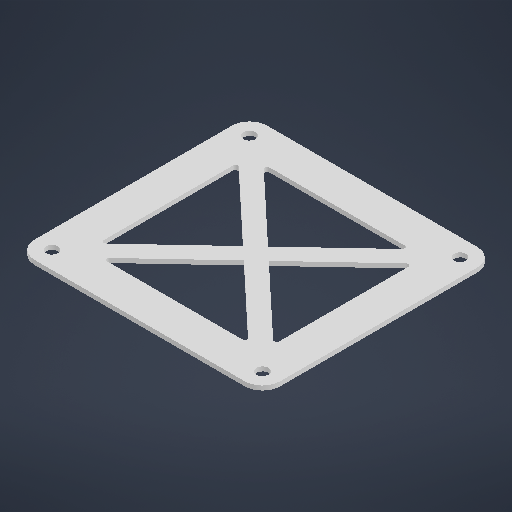
# Autodesk Inventor part: Hookcrossbrace
Saved by Autodesk Inventor 2025.2 (Build 292293000, 293)
## iProperties
Created: 2025-04-04
Part Number: Hookcrossbrace
Material: Generic
Document SubType Name: Modeling
Designer: Jahan
Density: 1 g/cm^3
Appearance: Default
Author: Jahan
Autodesk Inventor part; units mm, degrees
ref_plane "YZ Plane" through (0, 0, 0) normal (1, 0, 0) x (0, 1, 0)
ref_plane "XZ Plane" through (0, 0, 0) normal (0, 1, 0) x (-1, 0, 0)
ref_plane "XY Plane" through (0, 0, 0) normal (0, 0, 1) x (1, 0, 0)
sketch "Sketch1" plane through (0, 0, 0) normal (0, 1, 0) x (-1, 0, 0)
  circle A0 centre (-31.5089, -30.9076) radius 2.1844
  circle A1 centre (-31.5089, 40.6188) radius 2.1844
  circle A2 centre (44.6911, -30.9076) radius 2.1844
  circle A3 centre (44.6911, 40.6188) radius 2.1844
  circle A4 centre (44.6911, 40.6188) radius 6.35
  circle A5 centre (44.6911, -30.9076) radius 6.35
  circle A6 centre (-31.5089, -30.9076) radius 6.35
  circle A7 centre (-31.5089, 40.6188) radius 6.35
  line L0 (44.6911, 46.9688) -> (-31.5089, 46.9688)
  line L1 (-37.8589, 40.6188) -> (-37.8589, -30.9076)
  line L2 (-31.5089, -37.2576) -> (44.6911, -37.2576)
  line L3 (51.0411, -30.9076) -> (51.0411, 40.6188)
  line L4 (44.6911, 34.2688) -> (-31.5089, 34.2688)
  line L5 (-25.1589, 40.6188) -> (-25.1589, -30.9076)
  line L6 (-31.5089, -24.5576) -> (44.6911, -24.5576)
  line L7 (38.3411, 40.6188) -> (38.3411, -30.9076)
  line L8 (38.3411, 35.5878) -> (38.3411, 29.2378)
  line L9 (-25.1589, -24.5576) -> (-25.1589, -18.2076)
  line L10 (-25.1589, 34.2688) -> (-25.1589, 27.9188)
  line L11 (38.3411, -24.5576) -> (38.3411, -21.3826)
  line L12 (38.3411, -24.5576) -> (35.1661, -24.5576)
  line L13 (38.3411, 34.2688) -> (38.3411, 27.9188)
  line L14 (38.3411, -24.5576) -> (31.9911, -24.5576)
  circle A8 centre (-31.5089, 40.6188) radius 3.175
  circle A9 centre (44.6911, 40.6188) radius 3.175
  circle A10 centre (44.6911, -30.9076) radius 3.175
  circle A11 centre (-31.5089, -30.9076) radius 3.175
  line L15 (42.5182, 42.9337) -> (-33.6818, -28.5927)
  line L16 (46.8641, 38.3039) -> (-29.3359, -33.2225)
  line L17 (-29.3359, 42.9337) -> (46.8641, -28.5927)
  line L18 (-33.6818, 38.3039) -> (42.5182, -33.2225)
  arc A12 (31.6495, 32.7316) -> (31.041, 34.2688) centre (31.041, 33.3798) ccw
  arc A13 (38.3411, 28.2499) -> (36.8437, 28.8981) centre (37.4521, 28.2499) ccw
  arc A14 (36.8437, -19.1869) -> (38.3411, -18.5387) centre (37.4521, -18.5387) ccw
  arc A15 (31.041, -24.5576) -> (31.6495, -23.0204) centre (31.041, -23.6686) ccw
  arc A16 (-17.8588, 34.2688) -> (-18.4672, 32.7316) centre (-17.8588, 33.3798) ccw
  arc A17 (-23.6614, 28.8981) -> (-25.1589, 28.2499) centre (-24.2699, 28.2499) ccw
  arc A18 (-25.1589, -18.5387) -> (-23.6614, -19.1869) centre (-24.2699, -18.5387) ccw
  arc A19 (-18.4672, -23.0204) -> (-17.8588, -24.5576) centre (-17.8588, -23.6686) ccw
  point P0 (-25.1589, 30.3037)
  point P1 (1.952, 4.8556)
  point P2 (-25.1589, -20.5925)
  point P3 (-20.1048, 34.2688)
  point P4 (33.2871, 34.2688)
  point P5 (6.5911, 9.2102)
  point P6 (6.5911, 0.501)
  point P7 (-20.1048, -24.5576)
  point P8 (11.2303, 4.8556)
  point P9 (-25.1589, 28.2499)
  point P10 (-25.1589, -18.5387)
  dimension "d0" = 12.7
  dimension "d1" = 12.7
  dimension "d2" = 12.7
  dimension "d3" = 12.7
  dimension "d8" = 6.35
  dimension "d11" = 6.35
  dimension "d14" = 6.35
  dimension "d16" = 6.35
  dimension "d17" = 6.35
  dimension "d18" = 6.35
  dimension "d19" = 6.35
  dimension "d20" = 6.35
  dimension "d21" = 0.889
  dimension "d22" = 0.889
  dimension "d23" = 0.889
  dimension "d24" = 0.889
  dimension "d25" = 0.889
  dimension "d26" = 0.889
  dimension "d27" = 0.889
  dimension "d28" = 0.889
  constraints: 40 point on circle, 36 end point, 30 tangent, 24 point on line, 20 centre point, 8 coincident, 18 other
  measures "d0" diameter of A4
  measures "d1" diameter of A5
  measures "d2" diameter of A6
  measures "d3" diameter of A7
  measures "d8" distance of L9.start L9.end
  measures "d11" distance of L10.start L10.end
  measures "d14" distance of L13.start L13.end
  measures "d16" distance of L11.start L14.end
  measures "d17" diameter of A8
  measures "d18" diameter of A9
  measures "d19" diameter of A10
  measures "d20" diameter of A11
  measures "d21" radius of A12
  measures "d22" radius of A13
  measures "d23" radius of A14
  measures "d24" radius of A15
  measures "d25" radius of A16
  measures "d26" radius of A17
  measures "d27" radius of A18
  measures "d28" radius of A19
extrude "Extrusion1" add sketch "Sketch1" along normal blind 1.5875 contours A4 L16 A9 L15 | L3 A5 L6 L17 L7 L16 L4 A4 | A4 L7 L15 L4 L17 L5 A7 L0 | L4 L16 A4 | A5 L18 A10 L17 | A4 L15 L7 | A7 L17 A8 L18 | L16 L4 L7 L15 A4 | A4 L15 A9 L16 | L16 L7 L4 | A5 L17 L6 | L2 A6 L5 L16 L6 L18 L7 A5 | L7 L4 L15 | L5 L17 A7 | A7 L4 L18 L5 L15 L6 A6 L1 | A9 | L7 L16 L17 L15 L4 | L7 A13 L16 | L17 A10 L18 A5 | A5 L18 L7 L6 L17 | L6 L7 L17 | L7 L18 A5 | A6 L15 A11 L16 | L15 A12 L4 | L17 L5 L4 L18 A7 | A7 L18 A8 L17 | L17 L4 L5 | A7 L18 L4 | A10 | L7 L18 L6 | L6 L18 L16 L17 L7 | L17 A14 L7 | A6 L16 L5 | A8 | L5 L18 L4 | L4 L17 L15 L18 L5 | L4 A16 L17 | L6 L15 A6 | L16 L18 L15 L17 | L6 A15 L18 | L16 A11 L15 A6 | A6 L15 L6 L5 L16 | L5 L6 L16 | L18 A17 L5 | L15 L5 L6 | L16 L6 L5 L15 L18 | A11 | L16 A19 L6 | L5 A18 L15
body "Solid1"
